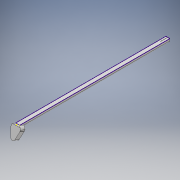
# Autodesk Inventor part: Bas du manche
Saved by Autodesk Inventor 2018.1 (Build 221171000, 171)
## iProperties
Created: 2019-11-08
Part Number: Bas du manche
Material: Générique
Document SubType Name: Modeling
Designer: tgremling1
Density: 1 g/cm^3
Appearance: Par défaut
Author: tgremling1
Autodesk Inventor part; units mm, degrees
ref_plane "YZ Plane" through (0, 0, 0) normal (1, 0, 0) x (0, 1, 0)
ref_plane "XZ Plane" through (0, 0, 0) normal (0, 1, 0) x (-1, 0, 0)
ref_plane "XY Plane" through (0, 0, 0) normal (0, 0, 1) x (1, 0, 0)
sketch "Esquisse1" plane through (0, 0, 0) normal (0, 1, 0) x (-1, 0, 0)
  line L0 (11, 11) -> (-11, 11)
  line L1 (-11, 11) -> (-11, -11)
  line L2 (-11, -11) -> (11, -11)
  line L3 (11, -11) -> (11, 11)
  point P0 (0, 0)
  constraints: 8 end point, 2 parallel, 1 horizontal, 1 perpendicular
extrude "Extrusion1" add sketch "Esquisse1" along normal blind 839.2
sketch "Esquisse2" plane through (11, 0, 11) normal (1, 0, 0) x (0, 0, -1)
  line L0 (0, 0) -> (22, 0) projected
  line L1 (0, 0) -> (10.2606, 28.1908)
  line L2 (10.2606, 28.1908) -> (76.0391, 4.2494)
  line L3 (10.2606, 28.1908) -> (80.2606, 28.1908) construction
  line L4 (76.0391, 4.2494) -> (65.7785, -23.9414)
  line L5 (65.7785, -23.9414) -> (0, 0)
  point P0 (11, 0)
  dimension "d7" = 30
  dimension "d8" = 70
  dimension "d9" = 20
  dimension "d10" = 30
  constraints: 10 end point, 2 perpendicular, 1 equal length, 1 horizontal
  measures "d7" distance of L0.start L1.end
  measures "d8" distance of L1.end L2.end
  measures "d9" angle of L2 L3
  measures "d10" distance of L2.end L4.end
extrude "Extrusion2" add sketch "Esquisse2" against normal blind 36 and the other way blind 14
fillet "Congé1" radius 14 2 edges at (25, 14.0954, 5.8697) (-25, 14.0954, 5.8697)
chamfer "Chanfrein1" distance 50 distance2 17 1 edges at (25, -9.846, -59.9088) measured on face at (25, 7.6212, -26.537)
chamfer "Chanfrein2" distance 50 distance2 17 1 edges at (-25, -9.846, -59.9088) measured on face at (-25, 7.6212, -26.537)
fillet "Congé2" radius 11 2 edges at (-8, -9.846, -59.9088) (8, -9.846, -59.9088)
fillet "Congé3" radius 5 2 edges at (-25, 7.255, -12.9242) (25, 7.255, -12.9242)
fillet "Congé4" radius 3 11 edges at (20.8995, 26.7883, -3.1138) (24.933, 21.3542, -18.044) (17.635, 13.9416, -38.4099) (6.5267, 4.9529, -63.106) (0, 4.2494, -65.0391) (-6.5267, 4.9529, -63.106) (-17.635, 13.9416, -38.4099) (-24.933, 21.3542, -18.044) (-25, 22.5178, -14.8469) (-20.8995, 26.7883, -3.1138) (25, 22.5178, -14.8469)
fillet "Congé5" radius 7 1 edges at (0, 0, 11)
fillet "Congé6" radius 10.5 2 edges at (11, 431.559, -11) (-11, 431.559, -11)
sketch "Esquisse5" plane through (0, 839.2, 0) normal (0, 1, 0) x (1, 0, 0)
  line L0 (-8, 0) -> (-8, -8)
  line L1 (8, 0) -> (8, -8)
  line L2 (8, -8) -> (-8, -8)
  arc A0 (8, 0.5) -> (0, 8) centre (-0.3442, -0.3838) ccw
  arc A1 (0, 8) -> (-8, 0.5) centre (-0.7644, 0.7987) ccw
  line L3 (8, -8) -> (8, 0.5)
  line L4 (-8, -8) -> (-8, 0.5)
  point P0 (0, 10.0144)
  point P1 (11, 0.5)
  constraints: 10 end point, 4 point on circle, 2 centre point
extrude "Extrusion3" cut sketch "Esquisse5" against normal blind 810
sketch "Esquisse6" plane through (-0.5, 23.918, -11) normal (0, 0, -1) x (-1, 0, 0)
  line L0 (-1, 775.282) -> (-0.0022, 775.282)
  line L1 (-8.5, 815.282) -> (7.5, 815.282) projected
  line L2 (0, 815.282) -> (-1, 815.282)
  line L3 (-1, 815.282) -> (-1, 775.282)
  line L4 (-1, 775.282) -> (0, 775.282)
  line L5 (0, 775.282) -> (0, 815.282)
  point P0 (-0.5, -23.918)
  point P1 (-10.5, 815.282)
  point P2 (9.5, 815.282)
  dimension "d37" = 1
  dimension "d38" = 40
  constraints: 10 end point, 2 parallel, 1 horizontal, 1 perpendicular, 1 point on line
  measures "d37" distance of L4.end L3.end
  measures "d38" distance of L3.end L2.end
extrude "Extrusion4" cut sketch "Esquisse6" against normal blind 30
sketch "Esquisse9" plane through (-11, 4.9015, 11) normal (0, 0, 1) x (1, 0, 0)
  line L0 (22, 0) -> (0, 0) projected
  line L1 (22, 0) -> (22, 834.2985) projected
  line L2 (0, 0) -> (22, 0)
  line L3 (22, 0) -> (22, 834.2985)
  line L4 (22, 834.2985) -> (0, 834.2985)
  line L5 (0, 834.2985) -> (0, 0)
  point P0 (11, -4.9015)
  constraints: 8 end point, 2 parallel, 1 horizontal, 1 perpendicular
